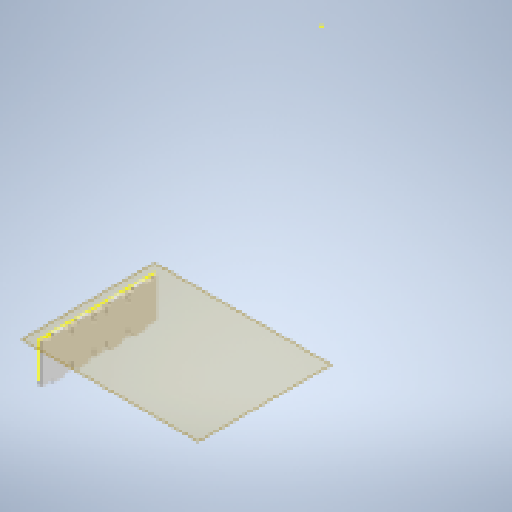
# Autodesk Inventor part: стенка
Saved by Autodesk Inventor 2024.2 (Build 282272000, 272)
## iProperties
Created: 2025-12-09
Part Number: стенка
Material: Типовые
Document SubType Name: Modeling
Designer: katya_notebook
Mass: 65.1748 g
Surface Area: 247.334 cm^2
Volume: 65.1748 cm^3
Density: 1 g/cm^3
Appearance: По умолчанию
Author: katya_notebook
Autodesk Inventor part; units mm, degrees
(part 1 of 2)
ref_plane "YZ Plane" through (0, 0, 0) normal (1, 0, 0) x (0, 1, 0)
ref_plane "XZ Plane" through (0, 0, 0) normal (0, 1, 0) x (-1, 0, 0)
ref_plane "РабПлоскость1" through (-475.2675, -216.9886, 379.0883) normal (0, 1, 0) x (-1, 0, 0)
sketch "Эскиз1" plane through (-475.2675, -216.9886, 379.0883) normal (0, 1, 0) x (-1, 0, 0)
  line L0 (135, 97.5) -> (129, 97.5)
  line L1 (129, 97.5) -> (129, -97.5)
  line L2 (129, -97.5) -> (135, -97.5)
  line L3 (135, -97.5) -> (135, 97.5)
  line L4 (135, -97.5) -> (135, 97.5) projected
  line L5 (68.1907, 97.5) -> (-80, 97.5) projected
  point P0 (-475.2675, -379.0883)
  point P1 (68.1907, -97.5)
  dimension "d0" = 0
  dimension "d1" = 6
  dimension "d3" = 0
  constraints: 8 end point, 2 parallel, 1 horizontal, 1 perpendicular, 1 vertical alignment
  measures "d0" horizontal extent of L3
  measures "d1" distance of L0.start L0.end
  measures "d3" distance between parallel lines of L0 L5
ref_plane "РабПлоскость2" through (-610.2675, -276.6936, 277.5883) normal (0, 1, 0) x (0, 0, 1)
extrude "Выдавливание1" add sketch "Эскиз1" against normal up to surface (59.705 mm away)
sketch "Эскиз2" plane through (-610.2675, -216.9886, 281.5883) normal (-1, 0, 0) x (0, 0, 1)
  line L0 (175, -4) -> (187, -4) projected
  line L1 (195, 0) -> (195, -59.705) projected
  line L2 (0, 0) -> (195, 0) projected
  line L3 (0, 0) -> (0, -59.705) projected
  point P0 (-281.5883, 216.9886)
  point P1 (195, -59.705)
  point P2 (0, -59.705)
  constraints: 2 other
sketch "Эскиз3" plane through (-610.2675, -276.6936, 281.5883) normal (-1, 0, 0) x (0, 0, 1)
  line L0 (195, 0) -> (0, 0) projected
  line L1 (175, 0) -> (155, 0)
  line L2 (155, 0) -> (155, -5)
  line L3 (155, -5) -> (175, -5)
  line L4 (175, -5) -> (175, 0)
  line L5 (195, 59.705) -> (195, 0) projected
  line L6 (135, 0) -> (115, 0)
  line L7 (115, 0) -> (115, -5)
  line L8 (115, -5) -> (135, -5)
  line L9 (135, -5) -> (135, 0)
  line L10 (20, 0) -> (40, 0)
  line L11 (40, 0) -> (40, -5)
  line L12 (40, -5) -> (20, -5)
  line L13 (20, -5) -> (20, 0)
  line L14 (60, 0) -> (80, 0)
  line L15 (80, 0) -> (80, -5)
  line L16 (80, -5) -> (60, -5)
  line L17 (60, -5) -> (60, 0)
  line L18 (97.5, 27.8525) -> (226.4185, 27.8525)
  line L19 (175, 55.705) -> (155, 55.705)
  line L20 (155, 55.705) -> (155, 60.705)
  line L21 (155, 60.705) -> (175, 60.705)
  line L22 (175, 60.705) -> (175, 55.705)
  line L23 (135, 55.705) -> (115, 55.705)
  line L24 (115, 55.705) -> (115, 60.705)
  line L25 (115, 60.705) -> (135, 60.705)
  line L26 (135, 60.705) -> (135, 55.705)
  line L27 (20, 55.705) -> (40, 55.705)
  line L28 (40, 55.705) -> (40, 60.705)
  line L29 (40, 60.705) -> (20, 60.705)
  line L30 (20, 60.705) -> (20, 55.705)
  line L31 (60, 55.705) -> (80, 55.705)
  line L32 (80, 55.705) -> (80, 60.705)
  line L33 (80, 60.705) -> (60, 60.705)
  line L34 (60, 60.705) -> (60, 55.705)
  point P0 (-281.5883, 276.6936)
  point P1 (40, 0)
  point P2 (80, 0)
  point P3 (115, 0)
  point P4 (155, 0)
  dimension "d0" = 0
  dimension "d8" = 5
  dimension "d9" = 20
  dimension "d10" = 20
  dimension "d11" = 20
  dimension "d12" = 20
  dimension "d13" = 5
  dimension "d14" = 20
  dimension "d15" = 20
  dimension "d16" = 20
  dimension "d17" = 20
  dimension "d43" = 5
  constraints: 66 end point, 16 symmetric about line, 8 parallel, 5 horizontal, 4 perpendicular, 4 point on line
  measures "d8" distance of L3.end L1.start
  measures "d9" distance of L2.end L3.end
  measures "d10" distance of L0.start L1.start
  measures "d11" distance of L7.end L8.end
  measures "d12" distance of L1.end L6.start
  measures "d13" distance of L10.end L11.end
  measures "d14" distance of L11.end L12.end
  measures "d15" distance of L10.start L0.end
  measures "d16" distance of L15.end L16.end
  measures "d17" distance of L14.start L10.end
  measures "d43" distance of L16.end L14.start
extrude "Выдавливание3" add sketch "Эскиз3" against normal blind 6
sketch "Эскиз4" plane through (-610.2675, -276.6936, 281.5883) normal (-1, 0, 0) x (0, 0, 1)
  point P0 (-281.5883, 276.6936)
sketch "Эскиз5" plane through (-610.2675, -276.6936, 281.5883) normal (-1, 0, 0) x (0, 0, 1)
  point P0 (-281.5883, 276.6936)
sketch "Эскиз7" plane through (-610.2675, -276.6936, 281.5883) normal (-1, 0, 0) x (0, 0, 1)
  line L0 (175, 55.705) -> (187, 55.705) projected
  line L1 (195, 59.705) -> (195, 0) projected
  line L2 (175, 59.705) -> (195, 59.705) projected
  line L3 (155, 55.705) -> (155, 59.705) projected
  line L4 (135, 55.705) -> (155, 55.705) projected
  line L5 (135, 59.705) -> (135, 55.705) projected
  line L6 (135, 59.705) -> (155, 59.705) projected
  line L7 (80, 55.705) -> (115, 55.705) projected
  line L8 (115, 55.705) -> (115, 59.705) projected
  line L9 (80, 59.705) -> (80, 55.705) projected
  line L10 (80, 59.705) -> (115, 59.705) projected
  line L11 (60, 55.705) -> (60, 59.705) projected
  line L12 (40, 55.705) -> (60, 55.705) projected
  line L13 (40, 59.705) -> (60, 59.705) projected
  line L14 (40, 59.705) -> (40, 55.705) projected
  line L15 (175, 55.705) -> (187, 55.705) projected
  line L16 (0, 59.705) -> (20, 59.705) projected
  line L17 (0, 59.705) -> (0, 0) projected
  point P0 (-281.5883, 276.6936)
  point P1 (195, 0)
  point P2 (0, 0)
  constraints: 2 other
extrude "Выдавливание5" cut sketch "Эскиз7" against normal blind 6
sketch "Эскиз8" plane through (-610.2675, -276.6936, 281.5883) normal (-1, 0, 0) x (0, 0, 1)
  line L0 (187, 59.705) -> (187, 55.705) projected
  line L1 (175, 59.705) -> (175, 55.705) projected
  line L2 (187, 55.705) -> (175, 55.705)
  line L3 (175, 55.705) -> (175, 59.705)
  line L4 (175, 59.705) -> (187, 59.705)
  line L5 (187, 59.705) -> (187, 55.705)
  line L6 (20, 55.705) -> (20, 59.705) projected
  line L7 (8, 55.705) -> (8, 59.705) projected
  line L8 (20, 55.705) -> (8, 55.705)
  line L9 (8, 55.705) -> (8, 59.705)
  line L10 (8, 59.705) -> (20, 59.705)
  line L11 (20, 59.705) -> (20, 55.705)
  point P0 (-281.5883, 276.6936)
  point P1 (8, 55.705)
  point P2 (20, 59.705)
  point P3 (175, 55.705)
  point P4 (187, 59.705)
  constraints: 16 end point, 4 parallel, 2 horizontal, 2 perpendicular
extrude "Выдавливание6" cut sketch "Эскиз8" against normal blind 10
sketch "Эскиз9" plane through (-610.2675, -276.6936, 281.5883) normal (-1, 0, 0) x (0, 0, 1)
  line L0 (163.4276, 22.0483) -> (4.2698, 22.0483) construction
  line L1 (4.2698, 22.0483) -> (4.2698, 35.3902) construction
  line L2 (4.2698, 35.3902) -> (163.4276, 35.3902) construction
  line L3 (163.4276, 35.3902) -> (163.4276, 22.0483) construction
  spline S0 degree 2 poles (156.433, 31.3837) (156.433, 32.4939) (157.9966, 34.0483) (159.1069, 34.0483) knots 0 0 0 1 2 2 2
  line L4 (159.1069, 34.0483) -> (159.9303, 34.0483)
  spline S1 degree 2 poles (159.9303, 34.0483) (161.0406, 34.0483) (162.5949, 32.4939) (162.5949, 31.3837) knots 0 0 0 1 2 2 2
  line L5 (162.5949, 31.3837) -> (162.5949, 24.7499)
  spline S2 degree 2 poles (162.5949, 24.7499) (162.5949, 23.6489) (161.0406, 22.0945) (159.9303, 22.0945) knots 0 0 0 1 2 2 2
  line L6 (159.9303, 22.0945) -> (159.1069, 22.0945)
  spline S3 degree 2 poles (159.1069, 22.0945) (157.9966, 22.0945) (156.433, 23.6489) (156.433, 24.7499) knots 0 0 0 1 2 2 2
  line L7 (156.433, 24.7499) -> (156.433, 31.3837)
  line L8 (157.6173, 31.3837) -> (157.6173, 24.7499)
  spline S4 degree 2 poles (157.6173, 24.7499) (157.6173, 24.1393) (158.4962, 23.2696) (159.1069, 23.2696) knots 0 0 0 1 2 2 2
  line L9 (159.1069, 23.2696) -> (159.9303, 23.2696)
  spline S5 degree 2 poles (159.9303, 23.2696) (160.5317, 23.2696) (161.4106, 24.1485) (161.4106, 24.7499) knots 0 0 0 1 2 2 2
  line L10 (161.4106, 24.7499) -> (161.4106, 31.3837)
  spline S6 degree 2 poles (161.4106, 31.3837) (161.4106, 31.9943) (160.5317, 32.8733) (159.9303, 32.8733) knots 0 0 0 1 2 2 2
  line L11 (159.9303, 32.8733) -> (159.1069, 32.8733)
  spline S7 degree 2 poles (159.1069, 32.8733) (158.4962, 32.8733) (157.6173, 32.0036) (157.6173, 31.3837) knots 0 0 0 1 2 2 2
  spline S8 degree 2 poles (149.6419, 33.4561) (149.6419, 34.0483) (150.2341, 34.0483) knots 0 0 0 1 1 1
  spline S9 degree 2 poles (150.2341, 34.0483) (150.8262, 34.0483) (150.8262, 33.4561) knots 0 0 0 1 1 1
  line L12 (150.8262, 33.4561) -> (150.8262, 26.5911)
  line L13 (150.8262, 26.5911) -> (152.251, 26.5911)
  line L14 (152.251, 26.5911) -> (153.8239, 33.6504)
  spline S10 degree 2 poles (153.8239, 33.6504) (153.9164, 34.0483) (154.379, 34.0483) knots 0 0 0 1 1 1
  spline S11 degree 2 poles (154.379, 34.0483) (154.9712, 34.0483) (154.9712, 33.4746) knots 0 0 0 1 1 1
  spline S12 degree 2 poles (154.9712, 33.4746) (154.9712, 33.4006) (154.9619, 33.3451) knots 0 0 0 1 1 1
  line L15 (154.9619, 33.3451) -> (153.2873, 25.8046)
  spline S13 degree 2 poles (153.2873, 25.8046) (153.1948, 25.416) (152.7229, 25.416) knots 0 0 0 1 1 1
  line L16 (152.7229, 25.416) -> (150.2341, 25.416)
  spline S14 degree 2 poles (150.2341, 25.416) (149.6419, 25.416) (149.6419, 25.9989) knots 0 0 0 1 1 1
  line L17 (149.6419, 25.9989) -> (149.6419, 33.4561)
  spline S15 degree 2 poles (142.8694, 33.4561) (142.8694, 34.0483) (143.4615, 34.0483) knots 0 0 0 1 1 1
  line L18 (143.4615, 34.0483) -> (146.3574, 34.0483)
  spline S16 degree 2 poles (146.3574, 34.0483) (147.1254, 34.0483) (148.1894, 32.975) (148.1894, 32.2164) knots 0 0 0 1 2 2 2
  line L19 (148.1894, 32.2164) -> (148.1894, 25.9989)
  spline S17 degree 2 poles (148.1894, 25.9989) (148.1894, 25.416) (147.5972, 25.416) knots 0 0 0 1 1 1
  spline S18 degree 2 poles (147.5972, 25.416) (147.0051, 25.416) (147.0051, 25.9989) knots 0 0 0 1 1 1
  line L20 (147.0051, 25.9989) -> (147.0051, 32.2071)
  spline S19 degree 2 poles (147.0051, 32.2071) (147.0051, 32.4847) (146.6165, 32.8733) (146.3574, 32.8733) knots 0 0 0 1 2 2 2
  line L21 (146.3574, 32.8733) -> (144.0537, 32.8733)
  line L22 (144.0537, 32.8733) -> (144.0537, 25.9989)
  spline S20 degree 2 poles (144.0537, 25.9989) (144.0537, 25.416) (143.4615, 25.416) knots 0 0 0 1 1 1
  spline S21 degree 2 poles (143.4615, 25.416) (142.8694, 25.416) (142.8694, 25.9989) knots 0 0 0 1 1 1
  line L23 (142.8694, 25.9989) -> (142.8694, 33.4561)
  spline S22 degree 2 poles (136.0783, 32.2164) (136.0783, 32.9658) (137.1516, 34.0483) (137.9288, 34.0483) knots 0 0 0 1 2 2 2
  line L24 (137.9288, 34.0483) -> (139.5664, 34.0483)
  spline S23 degree 2 poles (139.5664, 34.0483) (140.3436, 34.0483) (141.4168, 32.975) (141.4168, 32.2164) knots 0 0 0 1 2 2 2
  line L25 (141.4168, 32.2164) -> (141.4168, 23.9172)
  spline S24 degree 2 poles (141.4168, 23.9172) (141.4168, 23.066) (140.8432, 22.5664) knots 0 0 0 1 1 1
  spline S25 degree 2 poles (140.8432, 22.5664) (140.3343, 22.1038) (139.5849, 22.1038) knots 0 0 0 1 1 1
  spline S26 degree 2 poles (139.5849, 22.1038) (138.8447, 22.1038) (138.3266, 22.5664) knots 0 0 0 1 1 1
  spline S27 degree 2 poles (138.3266, 22.5664) (137.753, 23.0753) (137.753, 23.9265) knots 0 0 0 1 1 1
  spline S28 degree 2 poles (137.753, 23.9265) (137.753, 24.5741) (138.1786, 25.083) knots 0 0 0 1 1 1
  spline S29 degree 2 poles (138.1786, 25.083) (138.5301, 25.3698) (138.8817, 25.416) knots 0 0 0 1 1 1
  line L26 (138.8817, 25.416) -> (137.9288, 25.416)
  spline S30 degree 2 poles (137.9288, 25.416) (137.1516, 25.416) (136.0783, 26.4893) (136.0783, 27.2387) knots 0 0 0 1 2 2 2
  line L27 (136.0783, 27.2387) -> (136.0783, 32.2164)
  line L28 (137.2626, 32.2071) -> (137.2626, 27.2387)
  spline S31 degree 2 poles (137.2626, 27.2387) (137.2626, 26.9797) (137.6512, 26.5911) (137.9288, 26.5911) knots 0 0 0 1 2 2 2
  line L29 (137.9288, 26.5911) -> (139.5664, 26.5911)
  spline S32 degree 2 poles (139.5664, 26.5911) (139.8439, 26.5911) (140.2325, 26.9797) (140.2325, 27.2387) knots 0 0 0 1 2 2 2
  line L30 (140.2325, 27.2387) -> (140.2325, 32.2071)
  spline S33 degree 2 poles (140.2325, 32.2071) (140.2325, 32.4847) (139.8439, 32.8733) (139.5664, 32.8733) knots 0 0 0 1 2 2 2
  line L31 (139.5664, 32.8733) -> (137.9288, 32.8733)
  spline S34 degree 2 poles (137.9288, 32.8733) (137.6512, 32.8733) (137.2626, 32.4847) (137.2626, 32.2071) knots 0 0 0 1 2 2 2
  spline S35 degree 2 poles (138.928, 23.9265) (138.928, 23.6119) (139.3073, 23.2696) (139.5756, 23.2696) knots 0 0 0 1 2 2 2
  spline S36 degree 2 poles (139.5756, 23.2696) (139.8532, 23.2696) (140.1585, 23.4731) knots 0 0 0 1 1 1
  spline S37 degree 2 poles (140.1585, 23.4731) (140.2325, 23.6119) (140.2325, 23.9265) knots 0 0 0 1 1 1
  line L32 (140.2325, 23.9265) -> (140.2325, 25.4068)
  spline S38 degree 2 poles (140.2325, 25.4068) (139.6774, 24.9164) (139.187, 24.4168) knots 0 0 0 1 1 1
  spline S39 degree 2 poles (139.187, 24.4168) (138.928, 24.167) (138.928, 23.9265) knots 0 0 0 1 1 1
  spline S40 degree 2 poles (129.278, 26.0267) (129.278, 26.2395) (129.4353, 26.4153) knots 0 0 0 1 1 1
  spline S41 degree 2 poles (129.4353, 26.4153) (130.7306, 27.8401) (131.9611, 29.1446) knots 0 0 0 1 1 1
  line L33 (131.9611, 29.1446) -> (129.3891, 33.1508)
  spline S42 degree 2 poles (129.3891, 33.1508) (129.2965, 33.2989) (129.2965, 33.4561) knots 0 0 0 1 1 1
  spline S43 degree 2 poles (129.2965, 33.4561) (129.2965, 33.7059) (129.6666, 34.0483) (129.8979, 34.0483) knots 0 0 0 1 2 2 2
  spline S44 degree 2 poles (129.8979, 34.0483) (130.2032, 34.0483) (130.4068, 33.6412) knots 0 0 0 1 1 1
  line L34 (130.4068, 33.6412) -> (132.7383, 29.9403)
  spline S45 degree 2 poles (132.7383, 29.9403) (132.8123, 30.1439) (133.4415, 30.8378) knots 0 0 0 1 1 1
  line L35 (133.4415, 30.8378) -> (133.4415, 33.4561)
  spline S46 degree 2 poles (133.4415, 33.4561) (133.4415, 34.0483) (134.0336, 34.0483) knots 0 0 0 1 1 1
  spline S47 degree 2 poles (134.0336, 34.0483) (134.6258, 34.0483) (134.6258, 33.4561) knots 0 0 0 1 1 1
  line L36 (134.6258, 33.4561) -> (134.6258, 25.9989)
  spline S48 degree 2 poles (134.6258, 25.9989) (134.6258, 25.416) (134.0336, 25.416) knots 0 0 0 1 1 1
  spline S49 degree 2 poles (134.0336, 25.416) (133.4415, 25.416) (133.4415, 25.9989) knots 0 0 0 1 1 1
  line L37 (133.4415, 25.9989) -> (133.4415, 29.3482)
  line L38 (133.4415, 29.3482) -> (130.3605, 25.7121)
  spline S50 degree 2 poles (130.3605, 25.7121) (130.1292, 25.4345) (129.8887, 25.4345) knots 0 0 0 1 1 1
  spline S51 degree 2 poles (129.8887, 25.4345) (129.6389, 25.4345) (129.278, 25.7954) (129.278, 26.0267) knots 0 0 0 1 2 2 2
  spline S52 degree 2 poles (122.524, 32.2164) (122.524, 32.975) (123.5972, 34.0483) (124.3559, 34.0483) knots 0 0 0 1 2 2 2
  line L39 (124.3559, 34.0483) -> (126.012, 34.0483)
  spline S53 degree 2 poles (126.012, 34.0483) (126.78, 34.0483) (127.8439, 32.975) (127.8439, 32.2164) knots 0 0 0 1 2 2 2
  line L40 (127.8439, 32.2164) -> (127.8439, 27.2387)
  spline S54 degree 2 poles (127.8439, 27.2387) (127.8439, 26.4893) (126.7707, 25.416) (126.012, 25.416) knots 0 0 0 1 2 2 2
  line L41 (126.012, 25.416) -> (124.3559, 25.416)
  spline S55 degree 2 poles (124.3559, 25.416) (123.6065, 25.416) (122.524, 26.4985) (122.524, 27.2387) knots 0 0 0 1 2 2 2
  line L42 (122.524, 27.2387) -> (122.524, 32.2164)
  line L43 (123.7083, 32.2071) -> (123.7083, 27.2387)
  spline S56 degree 2 poles (123.7083, 27.2387) (123.7083, 26.9797) (124.0968, 26.5911) (124.3559, 26.5911) knots 0 0 0 1 2 2 2
  line L44 (124.3559, 26.5911) -> (126.012, 26.5911)
  spline S57 degree 2 poles (126.012, 26.5911) (126.2711, 26.5911) (126.6597, 26.9797) (126.6597, 27.2387) knots 0 0 0 1 2 2 2
  line L45 (126.6597, 27.2387) -> (126.6597, 32.2071)
  spline S58 degree 2 poles (126.6597, 32.2071) (126.6597, 32.4847) (126.2711, 32.8733) (126.012, 32.8733) knots 0 0 0 1 2 2 2
  line L46 (126.012, 32.8733) -> (124.3559, 32.8733)
  spline S59 degree 2 poles (124.3559, 32.8733) (124.0968, 32.8733) (123.7083, 32.4847) (123.7083, 32.2071) knots 0 0 0 1 2 2 2
  spline S60 degree 2 poles (115.7329, 32.2164) (115.7329, 32.9658) (116.8062, 34.0483) (117.5833, 34.0483) knots 0 0 0 1 2 2 2
  line L47 (117.5833, 34.0483) -> (119.221, 34.0483)
  spline S61 degree 2 poles (119.221, 34.0483) (119.9982, 34.0483) (121.0714, 32.975) (121.0714, 32.2164) knots 0 0 0 1 2 2 2
  line L48 (121.0714, 32.2164) -> (121.0714, 23.9172)
  spline S62 degree 2 poles (121.0714, 23.9172) (121.0714, 23.066) (120.4978, 22.5664) knots 0 0 0 1 1 1
  spline S63 degree 2 poles (120.4978, 22.5664) (119.9889, 22.1038) (119.2395, 22.1038) knots 0 0 0 1 1 1
  spline S64 degree 2 poles (119.2395, 22.1038) (118.4993, 22.1038) (117.9812, 22.5664) knots 0 0 0 1 1 1
  spline S65 degree 2 poles (117.9812, 22.5664) (117.4076, 23.0753) (117.4076, 23.9265) knots 0 0 0 1 1 1
  spline S66 degree 2 poles (117.4076, 23.9265) (117.4076, 24.5741) (117.8332, 25.083) knots 0 0 0 1 1 1
  spline S67 degree 2 poles (117.8332, 25.083) (118.1847, 25.3698) (118.5363, 25.416) knots 0 0 0 1 1 1
  line L49 (118.5363, 25.416) -> (117.5833, 25.416)
  spline S68 degree 2 poles (117.5833, 25.416) (116.8062, 25.416) (115.7329, 26.4893) (115.7329, 27.2387) knots 0 0 0 1 2 2 2
  line L50 (115.7329, 27.2387) -> (115.7329, 32.2164)
  line L51 (116.9172, 32.2071) -> (116.9172, 27.2387)
  spline S69 degree 2 poles (116.9172, 27.2387) (116.9172, 26.9797) (117.3058, 26.5911) (117.5833, 26.5911) knots 0 0 0 1 2 2 2
  line L52 (117.5833, 26.5911) -> (119.221, 26.5911)
  spline S70 degree 2 poles (119.221, 26.5911) (119.4985, 26.5911) (119.8871, 26.9797) (119.8871, 27.2387) knots 0 0 0 1 2 2 2
  line L53 (119.8871, 27.2387) -> (119.8871, 32.2071)
  spline S71 degree 2 poles (119.8871, 32.2071) (119.8871, 32.4847) (119.4985, 32.8733) (119.221, 32.8733) knots 0 0 0 1 2 2 2
  line L54 (119.221, 32.8733) -> (117.5833, 32.8733)
  spline S72 degree 2 poles (117.5833, 32.8733) (117.3058, 32.8733) (116.9172, 32.4847) (116.9172, 32.2071) knots 0 0 0 1 2 2 2
  spline S73 degree 2 poles (118.5826, 23.9265) (118.5826, 23.6119) (118.9619, 23.2696) (119.2302, 23.2696) knots 0 0 0 1 2 2 2
  spline S74 degree 2 poles (119.2302, 23.2696) (119.5078, 23.2696) (119.8131, 23.4731) knots 0 0 0 1 1 1
  spline S75 degree 2 poles (119.8131, 23.4731) (119.8871, 23.6119) (119.8871, 23.9265) knots 0 0 0 1 1 1
  line L55 (119.8871, 23.9265) -> (119.8871, 25.4068)
  spline S76 degree 2 poles (119.8871, 25.4068) (119.332, 24.9164) (118.8416, 24.4168) knots 0 0 0 1 1 1
  spline S77 degree 2 poles (118.8416, 24.4168) (118.5826, 24.167) (118.5826, 23.9265) knots 0 0 0 1 1 1
  spline S78 degree 2 poles (109.7838, 32.2164) (109.7838, 32.975) (110.8571, 34.0483) (111.625, 34.0483) knots 0 0 0 1 2 2 2
  line L56 (111.625, 34.0483) -> (113.6975, 34.0483)
  spline S79 degree 2 poles (113.6975, 34.0483) (114.2896, 34.0483) (114.2896, 33.4561) knots 0 0 0 1 1 1
  line L57 (114.2896, 33.4561) -> (114.2896, 25.9989)
  spline S80 degree 2 poles (114.2896, 25.9989) (114.2896, 25.416) (113.6975, 25.416) knots 0 0 0 1 1 1
  spline S81 degree 2 poles (113.6975, 25.416) (113.1053, 25.416) (113.1053, 25.9989) knots 0 0 0 1 1 1
  line L58 (113.1053, 25.9989) -> (113.1053, 29.1446)
  line L59 (113.1053, 29.1446) -> (111.6157, 29.1446)
  spline S82 degree 2 poles (111.6157, 29.1446) (110.8571, 29.1446) (109.7838, 30.2271) (109.7838, 30.9673) knots 0 0 0 1 2 2 2
  line L60 (109.7838, 30.9673) -> (109.7838, 32.2164)
  spline S83 degree 2 poles (108.1277, 33.4561) (108.1277, 34.0483) (108.7198, 34.0483) knots 0 0 0 1 1 1
  spline S84 degree 2 poles (108.7198, 34.0483) (109.312, 34.0483) (109.312, 33.4561) knots 0 0 0 1 1 1
  line L61 (109.312, 33.4561) -> (109.312, 25.9989)
  spline S85 degree 2 poles (109.312, 25.9989) (109.312, 25.416) (108.7198, 25.416) knots 0 0 0 1 1 1
  spline S86 degree 2 poles (108.7198, 25.416) (108.1277, 25.416) (108.1277, 25.9989) knots 0 0 0 1 1 1
  line L62 (108.1277, 25.9989) -> (108.1277, 33.4561)
  line L63 (110.9681, 32.2164) -> (110.9681, 30.9673)
  spline S87 degree 2 poles (110.9681, 30.9673) (110.9681, 30.7083) (111.3567, 30.3197) (111.625, 30.3197) knots 0 0 0 1 2 2 2
  line L64 (111.625, 30.3197) -> (113.1053, 30.3197)
  line L65 (113.1053, 30.3197) -> (113.1053, 32.8733)
  line L66 (113.1053, 32.8733) -> (111.625, 32.8733)
  spline S88 degree 2 poles (111.625, 32.8733) (111.3567, 32.8733) (110.9681, 32.4847) (110.9681, 32.2164) knots 0 0 0 1 2 2 2
  spline S89 degree 2 poles (101.3366, 33.4561) (101.3366, 34.0483) (101.9288, 34.0483) knots 0 0 0 1 1 1
  line L67 (101.9288, 34.0483) -> (104.8247, 34.0483)
  spline S90 degree 2 poles (104.8247, 34.0483) (105.5926, 34.0483) (106.6566, 32.975) (106.6566, 32.2071) knots 0 0 0 1 2 2 2
  line L68 (106.6566, 32.2071) -> (106.6566, 25.9897)
  spline S91 degree 2 poles (106.6566, 25.9897) (106.6566, 25.4068) (106.0645, 25.4068) knots 0 0 0 1 1 1
  spline S92 degree 2 poles (106.0645, 25.4068) (105.4723, 25.4068) (105.4723, 25.9897) knots 0 0 0 1 1 1
  line L69 (105.4723, 25.9897) -> (105.4723, 32.2071)
  spline S93 degree 2 poles (105.4723, 32.2071) (105.4723, 32.4847) (105.0837, 32.8733) (104.8247, 32.8733) knots 0 0 0 1 2 2 2
  line L70 (104.8247, 32.8733) -> (102.5209, 32.8733)
  line L71 (102.5209, 32.8733) -> (102.5209, 25.9897)
  spline S94 degree 2 poles (102.5209, 25.9897) (102.5209, 25.4068) (101.9288, 25.4068) knots 0 0 0 1 1 1
  spline S95 degree 2 poles (101.9288, 25.4068) (101.3366, 25.4068) (101.3366, 25.9897) knots 0 0 0 1 1 1
  line L72 (101.3366, 25.9897) -> (101.3366, 33.4561)
  line L73 (103.1778, 23.2696) -> (104.8154, 23.2696)
  spline S96 degree 2 poles (104.8154, 23.2696) (105.4076, 23.2696) (105.4076, 22.6774) knots 0 0 0 1 1 1
  spline S97 degree 2 poles (105.4076, 22.6774) (105.4076, 22.0945) (104.8154, 22.0945) knots 0 0 0 1 1 1
  line L74 (104.8154, 22.0945) -> (103.1778, 22.0945)
  spline S98 degree 2 poles (103.1778, 22.0945) (102.5857, 22.0945) (102.5857, 22.6774) knots 0 0 0 1 1 1
  spline S99 degree 2 poles (102.5857, 22.6774) (102.5857, 23.2696) (103.1778, 23.2696) knots 0 0 0 1 1 1
  spline S100 degree 2 poles (89.4384, 26.0267) (89.4384, 26.2395) (89.5957, 26.4153) knots 0 0 0 1 1 1
  spline S101 degree 2 poles (89.5957, 26.4153) (90.891, 27.8401) (92.1215, 29.1446) knots 0 0 0 1 1 1
  line L75 (92.1215, 29.1446) -> (89.5494, 33.1508)
  spline S102 degree 2 poles (89.5494, 33.1508) (89.4569, 33.2989) (89.4569, 33.4561) knots 0 0 0 1 1 1
  spline S103 degree 2 poles (89.4569, 33.4561) (89.4569, 33.7059) (89.827, 34.0483) (90.0583, 34.0483) knots 0 0 0 1 2 2 2
  spline S104 degree 2 poles (90.0583, 34.0483) (90.3636, 34.0483) (90.5672, 33.6412) knots 0 0 0 1 1 1
  line L76 (90.5672, 33.6412) -> (92.8987, 29.9403)
  spline S105 degree 2 poles (92.8987, 29.9403) (92.9727, 30.1439) (93.6018, 30.8378) knots 0 0 0 1 1 1
  line L77 (93.6018, 30.8378) -> (93.6018, 33.4561)
  spline S106 degree 2 poles (93.6018, 33.4561) (93.6018, 34.0483) (94.194, 34.0483) knots 0 0 0 1 1 1
  spline S107 degree 2 poles (94.194, 34.0483) (94.7861, 34.0483) (94.7861, 33.4561) knots 0 0 0 1 1 1
  line L78 (94.7861, 33.4561) -> (94.7861, 25.9989)
  spline S108 degree 2 poles (94.7861, 25.9989) (94.7861, 25.416) (94.194, 25.416) knots 0 0 0 1 1 1
  spline S109 degree 2 poles (94.194, 25.416) (93.6018, 25.416) (93.6018, 25.9989) knots 0 0 0 1 1 1
  line L79 (93.6018, 25.9989) -> (93.6018, 29.3482)
  line L80 (93.6018, 29.3482) -> (90.5209, 25.7121)
  spline S110 degree 2 poles (90.5209, 25.7121) (90.2896, 25.4345) (90.049, 25.4345) knots 0 0 0 1 1 1
  spline S111 degree 2 poles (90.049, 25.4345) (89.7992, 25.4345) (89.4384, 25.7954) (89.4384, 26.0267) knots 0 0 0 1 2 2 2
  spline S112 degree 2 poles (81.9164, 33.4654) (81.9164, 34.076) (82.4993, 34.076) knots 0 0 0 1 1 1
  spline S113 degree 2 poles (82.4993, 34.076) (82.9342, 34.076) (83.369, 33.4931) knots 0 0 0 1 1 1
  spline S114 degree 2 poles (83.369, 33.4931) (83.7761, 34.0483) (84.6088, 34.0483) knots 0 0 0 1 1 1
  line L81 (84.6088, 34.0483) -> (86.2649, 34.0483)
  spline S115 degree 2 poles (86.2649, 34.0483) (87.0328, 34.0483) (88.0968, 32.975) (88.0968, 32.2164) knots 0 0 0 1 2 2 2
  line L82 (88.0968, 32.2164) -> (88.0968, 27.2387)
  spline S116 degree 2 poles (88.0968, 27.2387) (88.0968, 26.4893) (87.0236, 25.416) (86.2649, 25.416) knots 0 0 0 1 2 2 2
  line L83 (86.2649, 25.416) -> (83.369, 25.416)
  spline S117 degree 2 poles (83.369, 25.416) (82.7769, 25.416) (82.7769, 25.9989) knots 0 0 0 1 1 1
  line L84 (82.7769, 25.9989) -> (82.7769, 32.2349)
  spline S118 degree 2 poles (82.7769, 32.2349) (82.7769, 32.7437) (82.3235, 32.9288) knots 0 0 0 1 1 1
  spline S119 degree 2 poles (82.3235, 32.9288) (81.9164, 33.0861) (81.9164, 33.4654) knots 0 0 0 1 1 1
  line L85 (83.9611, 32.2071) -> (83.9611, 26.5911)
  line L86 (83.9611, 26.5911) -> (86.2649, 26.5911)
  spline S120 degree 2 poles (86.2649, 26.5911) (86.524, 26.5911) (86.9126, 26.9797) (86.9126, 27.2387) knots 0 0 0 1 2 2 2
  line L87 (86.9126, 27.2387) -> (86.9126, 32.2071)
  spline S121 degree 2 poles (86.9126, 32.2071) (86.9126, 32.4847) (86.524, 32.8733) (86.2649, 32.8733) knots 0 0 0 1 2 2 2
  line L88 (86.2649, 32.8733) -> (84.6088, 32.8733)
  spline S122 degree 2 poles (84.6088, 32.8733) (84.3497, 32.8733) (83.9611, 32.4847) (83.9611, 32.2071) knots 0 0 0 1 2 2 2
  spline S123 degree 2 poles (75.9025, 32.2164) (75.9025, 32.9658) (76.9758, 34.0483) (77.7437, 34.0483) knots 0 0 0 1 2 2 2
  line L89 (77.7437, 34.0483) -> (79.3813, 34.0483)
  spline S124 degree 2 poles (79.3813, 34.0483) (80.1585, 34.0483) (81.2225, 32.975) (81.2225, 32.2164) knots 0 0 0 1 2 2 2
  line L90 (81.2225, 32.2164) -> (81.2225, 27.2387)
  spline S125 degree 2 poles (81.2225, 27.2387) (81.2225, 26.4893) (80.1585, 25.416) (79.3813, 25.416) knots 0 0 0 1 2 2 2
  line L91 (79.3813, 25.416) -> (78.4284, 25.416)
  line L92 (78.4284, 25.416) -> (80.9172, 23.1493)
  spline S126 degree 2 poles (80.9172, 23.1493) (81.278, 22.881) (81.278, 22.6127) knots 0 0 0 1 1 1
  spline S127 degree 2 poles (81.278, 22.6127) (81.278, 22.0945) (80.6304, 22.0945) knots 0 0 0 1 1 1
  line L93 (80.6304, 22.0945) -> (76.4947, 22.0945)
  spline S128 degree 2 poles (76.4947, 22.0945) (75.9025, 22.0945) (75.9025, 22.6774) knots 0 0 0 1 1 1
  spline S129 degree 2 poles (75.9025, 22.6774) (75.9025, 23.2696) (76.4947, 23.2696) knots 0 0 0 1 1 1
  line L94 (76.4947, 23.2696) -> (79.4369, 23.2696)
  line L95 (79.4369, 23.2696) -> (76.3651, 26.0729)
  spline S130 degree 2 poles (76.3651, 26.0729) (75.9025, 26.4893) (75.9025, 27.2387) knots 0 0 0 1 1 1
  line L96 (75.9025, 27.2387) -> (75.9025, 32.2164)
  line L97 (77.0868, 32.2071) -> (77.0868, 27.2387)
  spline S131 degree 2 poles (77.0868, 27.2387) (77.0868, 26.9797) (77.4754, 26.5911) (77.7437, 26.5911) knots 0 0 0 1 2 2 2
  line L98 (77.7437, 26.5911) -> (79.3813, 26.5911)
  spline S132 degree 2 poles (79.3813, 26.5911) (79.6497, 26.5911) (80.0382, 26.9797) (80.0382, 27.2387) knots 0 0 0 1 2 2 2
  line L99 (80.0382, 27.2387) -> (80.0382, 32.2071)
  spline S133 degree 2 poles (80.0382, 32.2071) (80.0382, 32.4847) (79.6497, 32.8733) (79.3813, 32.8733) knots 0 0 0 1 2 2 2
  line L100 (79.3813, 32.8733) -> (77.7437, 32.8733)
  spline S134 degree 2 poles (77.7437, 32.8733) (77.4754, 32.8733) (77.0868, 32.4847) (77.0868, 32.2071) knots 0 0 0 1 2 2 2
  line L101 (73.2564, 34.0575) -> (73.2564, 36.7776)
  spline S135 degree 2 poles (73.2564, 36.7776) (73.2564, 37.3698) (73.8486, 37.3698) knots 0 0 0 1 1 1
  spline S136 degree 2 poles (73.8486, 37.3698) (74.4407, 37.3698) (74.4407, 36.7776) knots 0 0 0 1 1 1
  line L102 (74.4407, 36.7776) -> (74.4407, 25.9989)
  spline S137 degree 2 poles (74.4407, 25.9989) (74.4407, 25.416) (73.8486, 25.416) knots 0 0 0 1 1 1
  line L103 (73.8486, 25.416) -> (70.9434, 25.416)
  spline S138 degree 2 poles (70.9434, 25.416) (70.194, 25.416) (69.1207, 26.4893) (69.1207, 27.2295) knots 0 0 0 1 2 2 2
  line L104 (69.1207, 27.2295) -> (69.1207, 32.2164)
  spline S139 degree 2 poles (69.1207, 32.2164) (69.1207, 32.9658) (70.194, 34.0575) (70.9434, 34.0575) knots 0 0 0 1 2 2 2
  line L105 (70.9434, 34.0575) -> (73.2564, 34.0575)
  line L106 (73.2564, 32.8825) -> (70.9434, 32.8825)
  spline S140 degree 2 poles (70.9434, 32.8825) (70.6843, 32.8825) (70.305, 32.4847) (70.305, 32.2164) knots 0 0 0 1 2 2 2
  line L107 (70.305, 32.2164) -> (70.305, 27.2387)
  spline S141 degree 2 poles (70.305, 27.2387) (70.305, 26.9797) (70.6936, 26.5911) (70.9434, 26.5911) knots 0 0 0 1 2 2 2
  line L108 (70.9434, 26.5911) -> (73.2564, 26.5911)
  line L109 (73.2564, 26.5911) -> (73.2564, 32.8825)
  spline S142 degree 2 poles (62.3389, 33.4561) (62.3389, 34.0483) (62.9311, 34.0483) knots 0 0 0 1 1 1
  line L110 (62.9311, 34.0483) -> (65.827, 34.0483)
  spline S143 degree 2 poles (65.827, 34.0483) (66.5949, 34.0483) (67.6589, 32.975) (67.6589, 32.2164) knots 0 0 0 1 2 2 2
  line L111 (67.6589, 32.2164) -> (67.6589, 25.9989)
  spline S144 degree 2 poles (67.6589, 25.9989) (67.6589, 25.416) (67.0668, 25.416) knots 0 0 0 1 1 1
  spline S145 degree 2 poles (67.0668, 25.416) (66.4746, 25.416) (66.4746, 25.9989) knots 0 0 0 1 1 1
  line L112 (66.4746, 25.9989) -> (66.4746, 32.2071)
  spline S146 degree 2 poles (66.4746, 32.2071) (66.4746, 32.4847) (66.086, 32.8733) (65.827, 32.8733) knots 0 0 0 1 2 2 2
  line L113 (65.827, 32.8733) -> (63.5232, 32.8733)
  line L114 (63.5232, 32.8733) -> (63.5232, 25.9989)
  spline S147 degree 2 poles (63.5232, 25.9989) (63.5232, 25.416) (62.9311, 25.416) knots 0 0 0 1 1 1
  spline S148 degree 2 poles (62.9311, 25.416) (62.3389, 25.416) (62.3389, 25.9989) knots 0 0 0 1 1 1
  line L115 (62.3389, 25.9989) -> (62.3389, 33.4561)
  spline S149 degree 2 poles (55.5571, 32.2164) (55.5571, 32.975) (56.6304, 34.0483) (57.389, 34.0483) knots 0 0 0 1 2 2 2
  line L116 (57.389, 34.0483) -> (59.0452, 34.0483)
  spline S150 degree 2 poles (59.0452, 34.0483) (59.8131, 34.0483) (60.8771, 32.975) (60.8771, 32.2164) knots 0 0 0 1 2 2 2
  line L117 (60.8771, 32.2164) -> (60.8771, 27.2387)
  spline S151 degree 2 poles (60.8771, 27.2387) (60.8771, 26.4893) (59.8039, 25.416) (59.0452, 25.416) knots 0 0 0 1 2 2 2
  line L118 (59.0452, 25.416) -> (57.389, 25.416)
  spline S152 degree 2 poles (57.389, 25.416) (56.6396, 25.416) (55.5571, 26.4985) (55.5571, 27.2387) knots 0 0 0 1 2 2 2
  line L119 (55.5571, 27.2387) -> (55.5571, 32.2164)
  line L120 (56.7414, 32.2071) -> (56.7414, 27.2387)
  spline S153 degree 2 poles (56.7414, 27.2387) (56.7414, 26.9797) (57.13, 26.5911) (57.389, 26.5911) knots 0 0 0 1 2 2 2
  line L121 (57.389, 26.5911) -> (59.0452, 26.5911)
  spline S154 degree 2 poles (59.0452, 26.5911) (59.3042, 26.5911) (59.6928, 26.9797) (59.6928, 27.2387) knots 0 0 0 1 2 2 2
  line L122 (59.6928, 27.2387) -> (59.6928, 32.2071)
  spline S155 degree 2 poles (59.6928, 32.2071) (59.6928, 32.4847) (59.3042, 32.8733) (59.0452, 32.8733) knots 0 0 0 1 2 2 2
  line L123 (59.0452, 32.8733) -> (57.389, 32.8733)
  spline S156 degree 2 poles (57.389, 32.8733) (57.13, 32.8733) (56.7414, 32.4847) (56.7414, 32.2071) knots 0 0 0 1 2 2 2
  spline S157 degree 2 poles (48.7661, 33.4561) (48.7661, 34.0483) (49.3582, 34.0483) knots 0 0 0 1 1 1
  spline S158 degree 2 poles (49.3582, 34.0483) (49.9503, 34.0483) (49.9503, 33.4561) knots 0 0 0 1 1 1
  line L124 (49.9503, 33.4561) -> (49.9503, 26.5911)
  line L125 (49.9503, 26.5911) -> (51.3752, 26.5911)
  line L126 (51.3752, 26.5911) -> (52.948, 33.6504)
  spline S159 degree 2 poles (52.948, 33.6504) (53.0406, 34.0483) (53.5032, 34.0483) knots 0 0 0 1 1 1
  spline S160 degree 2 poles (53.5032, 34.0483) (54.0953, 34.0483) (54.0953, 33.4746) knots 0 0 0 1 1 1
  spline S161 degree 2 poles (54.0953, 33.4746) (54.0953, 33.4006) (54.086, 33.3451) knots 0 0 0 1 1 1
  line L127 (54.086, 33.3451) -> (52.4114, 25.8046)
  spline S162 degree 2 poles (52.4114, 25.8046) (52.3189, 25.416) (51.847, 25.416) knots 0 0 0 1 1 1
  line L128 (51.847, 25.416) -> (49.3582, 25.416)
  spline S163 degree 2 poles (49.3582, 25.416) (48.7661, 25.416) (48.7661, 25.9989) knots 0 0 0 1 1 1
  line L129 (48.7661, 25.9989) -> (48.7661, 33.4561)
  line L130 (46.1292, 30.3197) -> (46.1292, 32.2164)
  spline S164 degree 2 poles (46.1292, 32.2164) (46.1292, 32.4939) (45.7499, 32.8733) (45.4908, 32.8733) knots 0 0 0 1 2 2 2
  line L131 (45.4908, 32.8733) -> (42.5949, 32.8733)
  spline S165 degree 2 poles (42.5949, 32.8733) (42.0028, 32.8733) (42.0028, 33.4561) knots 0 0 0 1 1 1
  spline S166 degree 2 poles (42.0028, 33.4561) (42.0028, 34.0483) (42.5949, 34.0483) knots 0 0 0 1 1 1
  line L132 (42.5949, 34.0483) -> (45.4908, 34.0483)
  spline S167 degree 2 poles (45.4908, 34.0483) (46.2587, 34.0483) (47.3135, 32.975) (47.3135, 32.2164) knots 0 0 0 1 2 2 2
  line L133 (47.3135, 32.2164) -> (47.3135, 27.2387)
  spline S168 degree 2 poles (47.3135, 27.2387) (47.3135, 26.4985) (46.2495, 25.416) (45.4908, 25.416) knots 0 0 0 1 2 2 2
  line L134 (45.4908, 25.416) -> (43.8254, 25.416)
  spline S169 degree 2 poles (43.8254, 25.416) (43.0668, 25.416) (41.9935, 26.4893) (41.9935, 27.248) knots 0 0 0 1 2 2 2
  line L135 (41.9935, 27.248) -> (41.9935, 29.7275)
  spline S170 degree 2 poles (41.9935, 29.7275) (41.9935, 30.3197) (42.5949, 30.3197) knots 0 0 0 1 1 1
  line L136 (42.5949, 30.3197) -> (46.1292, 30.3197)
  line L137 (46.1292, 29.1539) -> (43.1778, 29.1539)
  line L138 (43.1778, 29.1539) -> (43.1778, 27.248)
  spline S171 degree 2 poles (43.1778, 27.248) (43.1778, 26.9797) (43.5664, 26.5911) (43.8254, 26.5911) knots 0 0 0 1 2 2 2
  line L139 (43.8254, 26.5911) -> (45.4908, 26.5911)
  spline S172 degree 2 poles (45.4908, 26.5911) (45.7499, 26.5911) (46.1292, 26.9797) (46.1292, 27.248) knots 0 0 0 1 2 2 2
  line L140 (46.1292, 27.248) -> (46.1292, 29.1539)
  line L141 (37.2102, 26.5911) -> (39.3474, 26.5911)
  line L142 (39.3474, 26.5911) -> (39.3474, 33.4561)
  spline S173 degree 2 poles (39.3474, 33.4561) (39.3474, 34.0483) (39.9395, 34.0483) knots 0 0 0 1 1 1
  spline S174 degree 2 poles (39.9395, 34.0483) (40.5317, 34.0483) (40.5317, 33.4561) knots 0 0 0 1 1 1
  line L143 (40.5317, 33.4561) -> (40.5317, 25.9989)
  spline S175 degree 2 poles (40.5317, 25.9989) (40.5317, 25.416) (39.9395, 25.416) knots 0 0 0 1 1 1
  line L144 (39.9395, 25.416) -> (34.5456, 25.416)
  spline S176 degree 2 poles (34.5456, 25.416) (33.7869, 25.416) (32.7044, 26.4985) (32.7044, 27.2387) knots 0 0 0 1 2 2 2
  line L145 (32.7044, 27.2387) -> (32.7044, 33.4561)
  spline S177 degree 2 poles (32.7044, 33.4561) (32.7044, 34.0483) (33.2965, 34.0483) knots 0 0 0 1 1 1
  spline S178 degree 2 poles (33.2965, 34.0483) (33.8887, 34.0483) (33.8887, 33.4561) knots 0 0 0 1 1 1
  line L146 (33.8887, 33.4561) -> (33.8887, 27.248)
  spline S179 degree 2 poles (33.8887, 27.248) (33.8887, 26.9797) (34.2773, 26.5911) (34.5456, 26.5911) knots 0 0 0 1 2 2 2
  line L147 (34.5456, 26.5911) -> (36.0259, 26.5911)
  line L148 (36.0259, 26.5911) -> (36.0259, 33.4561)
  spline S180 degree 2 poles (36.0259, 33.4561) (36.0259, 34.0483) (36.618, 34.0483) knots 0 0 0 1 1 1
  spline S181 degree 2 poles (36.618, 34.0483) (37.2102, 34.0483) (37.2102, 33.4561) knots 0 0 0 1 1 1
  line L149 (37.2102, 33.4561) -> (37.2102, 26.5911)
  point P0 (-281.5883, 276.6936)
  constraints: 2 other
extrude "Выдавливание7" cut sketch "Эскиз9" against normal blind 1
sketch "Эскиз13" plane through (-610.2675, -276.6936, 281.5883) normal (-1, 0, 0) x (0, 0, 1)
  line L0 (155, -5) -> (175, -5) projected
  line L1 (175, -5) -> (155, -5)
  line L2 (155, -5) -> (155, -10.7721)
  line L3 (155, -10.7721) -> (175, -10.7721)
  line L4 (175, -10.7721) -> (175, -5)
  line L5 (115, -5) -> (135, -5) projected
  line L6 (135, -5) -> (115, -5)
  line L7 (115, -5) -> (115, -10.7721)
  line L8 (115, -10.7721) -> (135, -10.7721)
  line L9 (135, -10.7721) -> (135, -5)
  line L10 (80, -5) -> (60, -5)
  line L11 (60, -5) -> (60, -10.7721)
  line L12 (60, -10.7721) -> (80, -10.7721)
  line L13 (80, -10.7721) -> (80, -5)
  line L14 (40, -5) -> (40, 0) projected
  line L15 (40, -5) -> (20, -5)
  line L16 (20, -5) -> (20, -10.7721)
  line L17 (20, -10.7721) -> (40, -10.7721)
  line L18 (40, -10.7721) -> (40, -5)
  line L19 (175, -5) -> (175, 0) projected
  line L20 (175, 0) -> (195, 0)
  line L21 (195, 0) -> (195, -6.7721)
  line L22 (195, -6.7721) -> (175, -6.7721)
  line L23 (175, -6.7721) -> (175, 0)
  line L24 (155, 0) -> (155, -5) projected
  line L25 (155, 0) -> (135, 0)
  line L26 (135, 0) -> (135, -6.7721)
  line L27 (135, -6.7721) -> (155, -6.7721)
  line L28 (155, -6.7721) -> (155, 0)
  line L29 (115, 0) -> (80, 0)
  line L30 (80, 0) -> (80, -6.7721)
  line L31 (80, -6.7721) -> (115, -6.7721)
  line L32 (115, -6.7721) -> (115, 0)
  line L33 (60, 0) -> (40, 0)
  line L34 (40, 0) -> (40, -6.7721)
  line L35 (40, -6.7721) -> (60, -6.7721)
  line L36 (60, -6.7721) -> (60, 0)
  line L37 (20, 0) -> (0, 0)
  line L38 (0, 0) -> (0, -6.7721)
  line L39 (0, -6.7721) -> (20, -6.7721)
  line L40 (20, -6.7721) -> (20, 0)
  line L41 (0, 59.705) -> (0, 0) projected
  point P0 (-281.5883, 276.6936)
  point P1 (60, -5)
  point P2 (60, -5)
  point P3 (20, -6.7721)
  point P4 (60, -6.7721)
  point P5 (60, -5)
  point P6 (115, -6.7721)
  point P7 (155, -6.7721)
  constraints: 72 end point, 18 parallel, 10 point on line, 9 horizontal, 9 perpendicular
extrude "Выдавливание11" add sketch "Эскиз13" against normal blind 6 contours L0 L4 L3 L2 | L2 L27 L9 L26 L25 L24 | L9 L8 L7 L5 | L7 L31 L13 L30 L29 L32 | L13 L12 L11 L10 | L11 L35 L18 L14 L33 L36 | L18 L17 L16 L15 | L16 L39 L38 L37 L40
sketch "Эскиз6" plane through (-610.2675, -276.6936, 281.5883) normal (-1, 0, 0) x (0, 0, 1)
  line L0 (0, 59.705) -> (0, 0) construction
  line L1 (51.75, 61.7049) -> (48.25, 61.7049)
  line L2 (51.75, 43.7049) -> (51.75, 61.7049)
  line L3 (51.75, 43.7049) -> (48.25, 61.7049) construction
  line L4 (48.25, 43.7049) -> (51.75, 61.7049) construction
  line L5 (48.25, 61.7049) -> (48.25, 43.7049)
  line L6 (46.75, 54.2049) -> (46.75, 51.2049)
  line L7 (53.25, 54.2049) -> (46.75, 54.2049)
  line L8 (53.25, 51.2049) -> (53.25, 54.2049)
  line L9 (46.75, 51.2049) -> (53.25, 51.2049)
  line L10 (53.25, 52.7049) -> (46.75, 52.7049)
  line L11 (48.25, 43.7049) -> (51.75, 43.7049)
  line L12 (60, 55.7049) -> (60, 60.7049)
  line L13 (111.125, 54.2049) -> (104.625, 54.2049)
  line L14 (104.625, 54.2049) -> (104.625, 51.2049)
  line L15 (104.625, 51.2049) -> (111.125, 51.2049)
  line L16 (111.125, 51.2049) -> (111.125, 54.2049)
  line L17 (90.3751, 54.2049) -> (83.8751, 54.2049)
  line L18 (83.8751, 54.2049) -> (83.8751, 51.2049)
  line L19 (83.8751, 51.2049) -> (90.3751, 51.2049)
  line L20 (90.3751, 51.2049) -> (90.3751, 54.2049)
  line L21 (111.125, 52.7049) -> (104.625, 52.7049)
  line L22 (106.125, 49.7049) -> (109.625, 49.7049)
  line L23 (109.625, 49.7049) -> (109.625, 55.7049)
  line L24 (109.625, 55.7049) -> (106.125, 55.7049)
  line L25 (106.125, 55.7049) -> (106.125, 49.7049)
  line L26 (106.125, 49.7049) -> (109.625, 55.7049) construction
  line L27 (109.625, 49.7049) -> (106.125, 55.7049) construction
  line L28 (90.3751, 52.7049) -> (83.8751, 52.7049)
  line L29 (87.1251, 54.2049) -> (87.1251, 51.2049)
  line L30 (85.3751, 49.7049) -> (88.8751, 49.7049)
  line L31 (88.8751, 49.7049) -> (88.8751, 55.7049)
  line L32 (88.8751, 55.7049) -> (85.3751, 55.7049)
  line L33 (85.3751, 55.7049) -> (85.3751, 49.7049)
  line L34 (85.3751, 49.7049) -> (88.8751, 55.7049) construction
  line L35 (88.8751, 49.7049) -> (85.3751, 55.7049) construction
  line L36 (146.75, 61.7049) -> (143.25, 61.7049)
  line L37 (146.75, 43.7049) -> (146.75, 61.7049)
  line L38 (146.75, 43.7049) -> (143.25, 61.7049) construction
  line L39 (143.25, 43.7049) -> (146.75, 61.7049) construction
  line L40 (143.25, 61.7049) -> (143.25, 43.7049)
  line L41 (141.75, 54.2049) -> (141.75, 51.2049)
  line L42 (148.25, 54.2049) -> (141.75, 54.2049)
  line L43 (148.25, 51.2049) -> (148.25, 54.2049)
  line L44 (141.75, 51.2049) -> (148.25, 51.2049)
  line L45 (148.25, 52.7049) -> (141.75, 52.7049)
  line L46 (143.25, 43.7049) -> (146.75, 43.7049)
  line L47 (109.625, 49.7049) -> (106.125, 49.7049)
  line L48 (106.125, 49.7049) -> (106.125, 43.7049)
  line L49 (106.125, 43.7049) -> (109.625, 43.7049)
  line L50 (109.625, 43.7049) -> (109.625, 49.7049)
  line L51 (88.8751, 49.7049) -> (85.3751, 49.7049)
  line L52 (85.3751, 49.7049) -> (85.3751, 43.7049)
  line L53 (85.3751, 43.7049) -> (88.8751, 43.7049)
  line L54 (88.8751, 43.7049) -> (88.8751, 49.7049)
  line L55 (195, 59.705) -> (187, 59.705) projected
  line L56 (194.9984, -10.7631) -> (195, 24.4709)
  line L57 (195, 24.4709) -> (195, 59.705)
  line L58 (186.9984, -10.7722) -> (174.9984, -10.7722) projected
  ellipse E0 centre (186.9984, -10.7631) end of major axis (194.9984, -10.7631) minor radius 0.0091 (186.9984, -10.7722) -> (194.9984, -10.7631) ccw projected
  line L59 (195, 24.4709) -> (38.7239, 24.4709)
  line L60 (46.75, -5.263) -> (46.75, -2.263)
  line L61 (51.75, 5.237) -> (51.75, -12.763)
  line L62 (51.75, 5.237) -> (48.25, -12.763) construction
  line L63 (48.25, 5.237) -> (51.75, -12.763) construction
  line L64 (48.25, 5.237) -> (51.75, 5.237)
  line L65 (51.75, -12.763) -> (48.25, -12.763)
  line L66 (46.75, -2.263) -> (53.25, -2.263)
  line L67 (53.25, -2.263) -> (53.25, -5.263)
  line L68 (53.25, -5.263) -> (46.75, -5.263)
  line L69 (60, -6.763) -> (60, -11.763)
  line L70 (53.25, -3.763) -> (46.75, -3.763)
  line L71 (48.25, -12.763) -> (48.25, 5.237)
  line L72 (90.3751, -2.263) -> (90.3751, -5.263)
  line L73 (90.3751, -5.263) -> (83.8751, -5.263)
  line L74 (83.8751, -5.263) -> (83.8751, -2.263)
  line L75 (83.8751, -2.263) -> (90.3751, -2.263)
  line L76 (88.8751, 5.237) -> (88.8751, -0.763)
  line L77 (85.3751, -0.763) -> (85.3751, 5.237)
  line L78 (85.3751, 5.237) -> (88.8751, 5.237)
  line L79 (88.8751, -0.763) -> (88.8751, -6.763)
  line L80 (87.1251, -5.263) -> (87.1251, -2.263)
  line L81 (85.3751, -6.763) -> (85.3751, -0.763)
  line L82 (85.3751, -0.763) -> (88.8751, -6.763) construction
  line L83 (88.8751, -0.763) -> (85.3751, -6.763) construction
  line L84 (88.8751, -6.763) -> (85.3751, -6.763)
  line L85 (90.3751, -3.763) -> (83.8751, -3.763)
  line L86 (104.625, -2.263) -> (111.125, -2.263)
  line L87 (104.625, -5.263) -> (104.625, -2.263)
  line L88 (111.125, -2.263) -> (111.125, -5.263)
  line L89 (109.625, -0.763) -> (109.625, -6.763)
  line L90 (109.625, -6.763) -> (106.125, -6.763)
  line L91 (109.625, -0.763) -> (106.125, -6.763) construction
  line L92 (106.125, -6.763) -> (106.125, -0.763)
  line L93 (106.125, -0.763) -> (109.625, -6.763) construction
  line L94 (109.625, 5.237) -> (109.625, -0.763)
  line L95 (106.125, -0.763) -> (106.125, 5.237)
  line L96 (106.125, 5.237) -> (109.625, 5.237)
  line L97 (111.125, -3.763) -> (104.625, -3.763)
  line L98 (111.125, -5.263) -> (104.625, -5.263)
  line L99 (148.25, -5.263) -> (141.75, -5.263)
  line L100 (141.75, -5.263) -> (141.75, -2.263)
  line L101 (146.75, -12.763) -> (143.25, -12.763)
  line L102 (146.75, 5.237) -> (146.75, -12.763)
  line L103 (146.75, 5.237) -> (143.25, -12.763) construction
  line L104 (143.25, 5.237) -> (146.75, -12.763) construction
  line L105 (143.25, -12.763) -> (143.25, 5.237)
  line L106 (143.25, 5.237) -> (146.75, 5.237)
  line L107 (141.75, -2.263) -> (148.25, -2.263)
  line L108 (148.25, -3.763) -> (141.75, -3.763)
  line L109 (148.25, -2.263) -> (148.25, -5.263)
  point P0 (-281.5883, 276.6936)
  point P1 (50, 52.7049)
  point P2 (60, 58.2049)
  point P3 (115, 55.7049)
  point P4 (115, 58.2049)
  point P5 (107.875, 44.05)
  point P6 (107.875, 52.7049)
  point P7 (87.1251, 52.7049)
  point P8 (145, 52.7049)
  point P9 (143.25, 51.2049)
  point P10 (146.75, 51.2049)
  point P11 (146.75, 54.2049)
  point P12 (143.25, 54.2049)
  point P13 (51.75, 51.2049)
  point P14 (51.75, 54.2049)
  point P15 (48.25, 54.2049)
  point P16 (48.25, 51.2049)
  point P17 (109.625, 51.2049)
  point P18 (109.625, 54.2049)
  point P19 (106.125, 54.2049)
  point P20 (106.125, 51.2049)
  point P21 (106.125, 49.7049)
  point P22 (85.3751, 54.2049)
  point P23 (85.3751, 51.2049)
  point P24 (85.3751, 49.7049)
  point P25 (88.8751, 51.2049)
  point P26 (88.8751, 54.2049)
  point P27 (85.3751, 49.7049)
  point P28 (85.3751, 49.7049)
  point P29 (195, -6.7722)
  point P30 (0, -10.7631)
  point P31 (50, -3.763)
  point P32 (60, -9.263)
  point P33 (87.1251, -3.763)
  point P34 (107.875, -3.763)
  point P35 (145, -3.763)
  point P36 (48.25, -2.263)
  point P37 (48.25, -5.263)
  point P38 (51.75, -5.263)
  point P39 (51.75, -2.263)
  point P40 (85.3751, -5.263)
  point P41 (88.8751, -5.263)
  point P42 (106.125, -5.263)
  point P43 (109.625, -5.263)
  point P44 (109.625, -2.263)
  point P45 (106.125, -0.763)
  point P46 (106.125, -2.263)
  point P47 (146.75, -2.263)
  point P48 (143.25, -2.263)
  point P49 (143.25, -5.263)
  point P50 (146.75, -5.263)
  constraints: 214 end point, 56 symmetric about line, 1 equal length, 1 horizontal, 1 vertical, 2 other